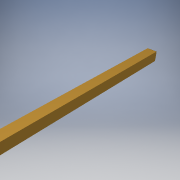
# Autodesk Inventor part: Pin male header straight - single
Saved by Autodesk Inventor 2017 (Build 210142000, 142)
## iProperties
Created: 2017-09-07
Part Number: Pin male header straight - single
Material: Brass, Soft Yellow
Document SubType Name: Modeling
Designer: denoqs
Density: 8.47 g/cm^3
Appearance: Brass - Satin
Author: denoqs
Autodesk Inventor part; units mm, degrees
ref_plane "YZ Plane" through (0, 0, 0) normal (1, 0, 0) x (0, 1, 0)
ref_plane "XZ Plane" through (0, 0, 0) normal (0, 1, 0) x (-1, 0, 0)
ref_plane "XY Plane" through (0, 0, 0) normal (0, 0, 1) x (1, 0, 0)
sketch "Sketch1" plane through (0, 0, 0) normal (0, 1, 0) x (-1, 0, 0)
  line L0 (0.325, 0.325) -> (-0.325, 0.325)
  line L1 (-0.325, 0.325) -> (-0.325, -0.325)
  line L2 (-0.325, -0.325) -> (0.325, -0.325)
  line L3 (0.325, -0.325) -> (0.325, 0.325)
  point P0 (0, 0)
  point P1 (0, -0.325)
  point P2 (-0.325, 0)
  dimension "d0" = 0.65
  dimension "d1" = 0.65
  constraints: 8 end point, 2 midpoint, 2 parallel, 1 horizontal, 1 horizontal alignment, 1 perpendicular, 1 vertical alignment
  measures "d0" distance of L0.end L1.end
  measures "d1" distance of L1.end L2.end
extrude "Extrusion1" add sketch "Sketch1" along normal blind 11.2
chamfer "Chamfer1" distance 0.1 distance2 0.2 1 edges at (0.325, 0, 0) measured on face at (0.1083, 0, 0.1083)
chamfer "Chamfer2" distance 0.1 distance2 0.2 1 edges at (-0.325, 0, 0) measured on face at (0.0417, 0, 0.1083)
chamfer "Chamfer3" distance 0.1 distance2 0.2 1 edges at (0, 0, 0.325) measured on face at (0.075, 0, 0.1083)
chamfer "Chamfer4" distance 0.1 distance2 0.2 1 edges at (0, 0, -0.325) measured on face at (0.075, 0, 0.0417)
chamfer "Chamfer5" distance 0.1 distance2 0.2 1 edges at (0.325, 11.2, 0) measured on face at (0.1083, 11.2, 0.1083)
chamfer "Chamfer6" distance 0.1 distance2 0.2 1 edges at (-0.05, 11.2, 0.325) measured on face at (0.0417, 11.2, 0.1083)
chamfer "Chamfer7" distance 0.1 distance2 0.2 1 edges at (-0.325, 11.2, -0.05) measured on face at (-0.1417, 11.2, -0.1417)
chamfer "Chamfer8" distance 0.1 distance2 0.2 1 edges at (0, 11.2, -0.325) measured on face at (-0.075, 11.2, -0.1417)
equation "\"d1\" = d0"
body "Solid1"
